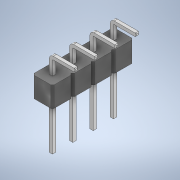
# Autodesk Inventor part: Part7
Saved by Autodesk Inventor 2021 (Build 250183000, 183)
## iProperties
Created: 2023-04-17
Part Number: Part7
Material: Generic
Document SubType Name: Modeling
Designer: stepa
Density: 1 g/cm^3
Appearance: Default
Author: stepa
Autodesk Inventor part; units mm, degrees
ref_plane "YZ Plane" through (0, 0, 0) normal (1, 0, 0) x (0, 1, 0)
ref_plane "XZ Plane" through (0, 0, 0) normal (0, 1, 0) x (-1, 0, 0)
sketch "Sketch1" plane through (0, 0, 0) normal (0, 1, 0) x (-1, 0, 0)
  line L0 (1.3038, 10.4024) -> (-0.7962, 10.4024)
  line L1 (-0.9962, 10.2024) -> (-0.9962, 8.1024)
  line L2 (-0.7962, 7.9024) -> (1.3038, 7.9024)
  line L3 (1.5038, 8.1024) -> (1.5038, 10.2024)
  line L4 (1.5038, 10.4024) -> (-0.9962, 7.9024) construction
  line L5 (-0.9962, 10.4024) -> (1.5038, 7.9024) construction
  line L6 (1.3038, 10.4024) -> (1.5038, 10.2024)
  line L7 (1.5038, 8.1024) -> (1.3038, 7.9024)
  line L8 (-0.9962, 8.1024) -> (-0.7962, 7.9024)
  line L9 (-0.9962, 10.2024) -> (-0.7962, 10.4024)
  line L10 (1.3038, 7.8624) -> (1.5038, 7.6624)
  line L11 (1.3038, 7.8624) -> (-0.7962, 7.8624)
  line L12 (-0.9962, 7.6624) -> (-0.7962, 7.8624)
  line L13 (1.5038, 5.5624) -> (1.5038, 7.6624)
  line L14 (1.5038, 5.5624) -> (1.3038, 5.3624)
  line L15 (-0.9962, 7.6624) -> (-0.9962, 5.5624)
  line L16 (-0.7962, 5.3624) -> (1.3038, 5.3624)
  line L17 (-0.9962, 5.5624) -> (-0.7962, 5.3624)
  line L18 (-0.9962, 7.8624) -> (1.5038, 5.3624) construction
  line L19 (1.5038, 7.8624) -> (-0.9962, 5.3624) construction
  line L20 (1.3038, 5.3224) -> (1.5038, 5.1224)
  line L21 (1.3038, 5.3224) -> (-0.7962, 5.3224)
  line L22 (-0.9962, 5.1224) -> (-0.7962, 5.3224)
  line L23 (1.5038, 3.0224) -> (1.5038, 5.1224)
  line L24 (1.5038, 3.0224) -> (1.3038, 2.8224)
  line L25 (-0.9962, 5.1224) -> (-0.9962, 3.0224)
  line L26 (-0.7962, 2.8224) -> (1.3038, 2.8224)
  line L27 (-0.9962, 3.0224) -> (-0.7962, 2.8224)
  line L28 (-0.9962, 5.3224) -> (1.5038, 2.8224) construction
  line L29 (1.5038, 5.3224) -> (-0.9962, 2.8224) construction
  line L30 (1.3038, 2.7824) -> (1.5038, 2.5824)
  line L31 (1.3038, 2.7824) -> (-0.7962, 2.7824)
  line L32 (-0.9962, 2.5824) -> (-0.7962, 2.7824)
  line L33 (1.5038, 0.4824) -> (1.5038, 2.5824)
  line L34 (1.5038, 0.4824) -> (1.3038, 0.2824)
  line L35 (-0.9962, 2.5824) -> (-0.9962, 0.4824)
  line L36 (-0.7962, 0.2824) -> (1.3038, 0.2824)
  line L37 (-0.9962, 0.4824) -> (-0.7962, 0.2824)
  line L38 (-0.9962, 2.7824) -> (1.5038, 0.2824) construction
  line L39 (1.5038, 2.7824) -> (-0.9962, 0.2824) construction
  line L40 (1.3038, 7.9024) -> (1.3038, 2.7824)
  line L41 (-0.7962, 2.7824) -> (-0.7962, 7.9024)
  point P0 (0, 0)
  point P1 (0.2538, 9.1524)
  point P2 (0.2538, 6.6124)
  point P3 (0.2538, 4.0724)
  point P4 (0.2538, 1.5324)
  dimension "d0" = 2.5
  dimension "d1" = 2.5
  dimension "d2" = 0.2
  dimension "d3" = 0.2
  dimension "d4" = 0.2
  dimension "d5" = 0.2
  dimension "d6" = 0.2
  dimension "d7" = 0.2
  dimension "d8" = 0.2
  dimension "d9" = 0.2
  dimension "d12" = 2.54
  constraints: 84 end point, 32 point on line, 8 midpoint, 2 parallel, 1 collinear, 1 horizontal, 1 perpendicular, 1 vertical, 68 other
  measures "d0" distance of L5.end L4.start
  measures "d1" distance of L4.end L5.end
  measures "d2" distance of L0.start L4.start
  measures "d3" distance of L3.end L4.start
  measures "d4" distance of L3.start L5.end
  measures "d5" distance of L2.end L5.end
  measures "d6" distance of L1.end L4.end
  measures "d7" distance of L2.start L4.end
  measures "d8" distance of L1.start L5.start
  measures "d9" distance of L0.end L5.start
  measures "d12" distance of L0.start L10.start
extrude "Extrusion1" add sketch "Sketch1" along normal blind 2.54
sketch "Sketch2" plane through (0, 2.54, 0) normal (0, 1, 0) x (1, 0, 0)
  line L0 (-1.5038, -8.1024) -> (-1.3038, -7.9024) projected
  line L1 (-1.3038, -7.9024) -> (-1.3038, -7.8624) projected
  line L2 (-1.3038, -7.8624) -> (-1.5038, -7.6624) projected
  line L3 (-1.5038, -7.6624) -> (-1.5038, -5.5624) projected
  line L4 (-1.5038, -5.5624) -> (-1.3038, -5.3624) projected
  line L5 (-1.3038, -5.3624) -> (-1.3038, -5.3224) projected
  line L6 (-1.3038, -5.3224) -> (-1.5038, -5.1224) projected
  line L7 (-1.5038, -5.1224) -> (-1.5038, -3.0224) projected
  line L8 (-1.5038, -3.0224) -> (-1.3038, -2.8224) projected
  line L9 (-1.3038, -2.8224) -> (-1.3038, -2.7824) projected
  line L10 (-1.3038, -2.7824) -> (-1.5038, -2.5824) projected
  line L11 (-1.5038, -2.5824) -> (-1.5038, -0.4824) projected
  line L12 (-1.5038, -0.4824) -> (-1.3038, -0.2824) projected
  line L13 (-1.3038, -0.2824) -> (0.7962, -0.2824) projected
  line L14 (0.7962, -0.2824) -> (0.9962, -0.4824) projected
  line L15 (0.9962, -0.4824) -> (0.9962, -2.5824) projected
  line L16 (0.9962, -2.5824) -> (0.7962, -2.7824) projected
  line L17 (0.7962, -2.7824) -> (0.7962, -2.8224) projected
  line L18 (0.7962, -2.8224) -> (0.9962, -3.0224) projected
  line L19 (0.9962, -3.0224) -> (0.9962, -5.1224) projected
  line L20 (0.9962, -5.1224) -> (0.7962, -5.3224) projected
  line L21 (0.7962, -5.3224) -> (0.7962, -5.3624) projected
  line L22 (0.7962, -5.3624) -> (0.9962, -5.5624) projected
  line L23 (0.9962, -5.5624) -> (0.9962, -7.6624) projected
  line L24 (0.9962, -7.6624) -> (0.7962, -7.8624) projected
  line L25 (0.7962, -7.8624) -> (0.7962, -7.9024) projected
  line L26 (0.7962, -7.9024) -> (0.9962, -8.1024) projected
  line L27 (0.9962, -8.1024) -> (0.9962, -10.2024) projected
  line L28 (0.9962, -10.2024) -> (0.7962, -10.4024) projected
  line L29 (0.7962, -10.4024) -> (-1.3038, -10.4024) projected
  line L30 (-1.3038, -10.4024) -> (-1.5038, -10.2024) projected
  line L31 (-1.5038, -10.2024) -> (-1.5038, -8.1024) projected
  point P0 (0, 0)
  point P1 (-0.2538, -1.5324)
  point P2 (-0.2538, -1.5324)
  point P3 (-0.2538, -4.0724)
  point P4 (-0.2538, -6.6124)
  point P5 (-0.2538, -9.1524)
  constraints: 1 coincident
ref_plane "Work Plane1" through (2.7462, 4.54, 9.1524) normal (1, 0, 0) x (0, 0, -1)
sketch "Sketch3" plane through (2.7462, 4.54, 9.1524) normal (1, 0, 0) x (0, 0, -1)
  line L0 (-0.2, 0.2) -> (0.2, 0.2)
  line L1 (0.2, 0.2) -> (0.2, -0.2)
  line L2 (0.2, -0.2) -> (-0.2, -0.2)
  line L3 (-0.2, -0.2) -> (-0.2, 0.2)
  line L4 (-0.2, 0.2) -> (0.2, -0.2) construction
  line L5 (0.2, 0.2) -> (-0.2, -0.2) construction
  line L6 (2.34, 0.2) -> (2.74, 0.2)
  line L7 (2.74, 0.2) -> (2.74, -0.2)
  line L8 (2.74, -0.2) -> (2.34, -0.2)
  line L9 (2.34, -0.2) -> (2.34, 0.2)
  line L10 (2.34, 0.2) -> (2.74, -0.2) construction
  line L11 (2.74, 0.2) -> (2.34, -0.2) construction
  line L12 (4.88, 0.2) -> (5.28, 0.2)
  line L13 (5.28, 0.2) -> (5.28, -0.2)
  line L14 (5.28, -0.2) -> (4.88, -0.2)
  line L15 (4.88, -0.2) -> (4.88, 0.2)
  line L16 (4.88, 0.2) -> (5.28, -0.2) construction
  line L17 (5.28, 0.2) -> (4.88, -0.2) construction
  line L18 (7.42, 0.2) -> (7.82, 0.2)
  line L19 (7.82, 0.2) -> (7.82, -0.2)
  line L20 (7.82, -0.2) -> (7.42, -0.2)
  line L21 (7.42, -0.2) -> (7.42, 0.2)
  line L22 (7.42, 0.2) -> (7.82, -0.2) construction
  line L23 (7.82, 0.2) -> (7.42, -0.2) construction
  point P0 (9.1524, -4.54)
  point P1 (0, 0)
  point P2 (2.54, 0)
  point P3 (5.08, 0)
  point P4 (7.62, 0)
  dimension "d32" = 0.4
  dimension "d33" = 0.4
  dimension "d36" = 2.54
  constraints: 48 end point, 8 midpoint, 2 horizontal, 2 parallel, 1 collinear, 1 perpendicular, 32 other
  measures "d32" distance of L0.end L1.end
  measures "d33" distance of L1.end L2.end
  measures "d36" distance of L0.start L6.start
sketch3d "3D Sketch2"
  line L0 (2.7462, 4.54, 9.1524) -> (0.0462, 4.54, 9.1524)
  arc A0 (0.0462, 4.54, 9.1524) -> (-0.2538, 4.24, 9.1524) centre (0.0462, 4.24, 9.1524) ccw
  line L1 (-0.2538, 4.24, 9.1524) -> (-0.2538, 2.54, 9.1524)
  dimension "d19" = 2
  dimension "d20" = 3
  dimension "d21" = 2
  dimension "d22" = 3
  dimension "d23" = 2
  dimension "d24" = 3
  dimension "d25" = 2
  dimension "d27" = 3
  dimension "d28" = 0.3
  dimension "d29" = 0.3
  dimension "d30" = 0.3
  dimension "d31" = 0.3
sweep "Sweep1" add profiles "Sketch3" path "3D Sketch2"
chamfer "Chamfer1" distance 0.1 angle 45 16 edges at (2.7462, 4.54, 9.3524) (2.7462, 4.74, 9.1524) (2.7462, 4.34, 9.1524) (2.7462, 4.54, 8.9524) (2.7462, 4.54, 6.8124) (2.7462, 4.74, 6.6124) (2.7462, 4.54, 6.4124) (2.7462, 4.34, 6.6124) (2.7462, 4.54, 4.2724) (2.7462, 4.74, 4.0724) (2.7462, 4.54, 3.8724) (2.7462, 4.34, 4.0724) (2.7462, 4.54, 1.7324) (2.7462, 4.74, 1.5324) (2.7462, 4.54, 1.3324) (2.7462, 4.34, 1.5324)
sketch "Sketch4" plane through (0, 0, 0) normal (0, -1, 0) x (1, 0, 0)
  line L0 (-1.3038, 7.9024) -> (-1.5038, 8.1024) projected
  line L1 (-1.5038, 8.1024) -> (-1.5038, 10.2024) projected
  line L2 (-1.5038, 10.2024) -> (-1.3038, 10.4024) projected
  line L3 (-1.3038, 10.4024) -> (0.7962, 10.4024) projected
  line L4 (0.7962, 10.4024) -> (0.9962, 10.2024) projected
  line L5 (0.9962, 10.2024) -> (0.9962, 8.1024) projected
  line L6 (0.9962, 8.1024) -> (0.7962, 7.9024) projected
  line L7 (0.7962, 7.9024) -> (0.7962, 7.8624) projected
  line L8 (0.7962, 7.8624) -> (0.9962, 7.6624) projected
  line L9 (0.9962, 7.6624) -> (0.9962, 5.5624) projected
  line L10 (0.9962, 5.5624) -> (0.7962, 5.3624) projected
  line L11 (0.7962, 5.3624) -> (0.7962, 5.3224) projected
  line L12 (0.7962, 5.3224) -> (0.9962, 5.1224) projected
  line L13 (0.9962, 5.1224) -> (0.9962, 3.0224) projected
  line L14 (0.9962, 3.0224) -> (0.7962, 2.8224) projected
  line L15 (0.7962, 2.8224) -> (0.7962, 2.7824) projected
  line L16 (0.7962, 2.7824) -> (0.9962, 2.5824) projected
  line L17 (0.9962, 2.5824) -> (0.9962, 0.4824) projected
  line L18 (0.9962, 0.4824) -> (0.7962, 0.2824) projected
  line L19 (0.7962, 0.2824) -> (-1.3038, 0.2824) projected
  line L20 (-1.3038, 0.2824) -> (-1.5038, 0.4824) projected
  line L21 (-1.5038, 0.4824) -> (-1.5038, 2.5824) projected
  line L22 (-1.5038, 2.5824) -> (-1.3038, 2.7824) projected
  line L23 (-1.3038, 2.7824) -> (-1.3038, 2.8224) projected
  line L24 (-1.3038, 2.8224) -> (-1.5038, 3.0224) projected
  line L25 (-1.5038, 3.0224) -> (-1.5038, 5.1224) projected
  line L26 (-1.5038, 5.1224) -> (-1.3038, 5.3224) projected
  line L27 (-1.3038, 5.3224) -> (-1.3038, 5.3624) projected
  line L28 (-1.3038, 5.3624) -> (-1.5038, 5.5624) projected
  line L29 (-1.5038, 5.5624) -> (-1.5038, 7.6624) projected
  line L30 (-1.5038, 7.6624) -> (-1.3038, 7.8624) projected
  line L31 (-1.3038, 7.8624) -> (-1.3038, 7.9024) projected
  line L32 (-0.0538, 1.3324) -> (-0.0538, 1.7324) projected
  line L33 (-0.4538, 1.3324) -> (-0.0538, 1.3324) projected
  line L34 (-0.4538, 1.7324) -> (-0.4538, 1.3324) projected
  line L35 (-0.0538, 1.7324) -> (-0.4538, 1.7324) projected
  line L36 (-0.4538, 3.8724) -> (-0.0538, 3.8724) projected
  line L37 (-1.5038, 8.1024) -> (-1.5038, 10.2024) projected
  line L38 (-1.3038, 7.9024) -> (-1.5038, 8.1024) projected
  line L39 (-1.3038, 7.8624) -> (-1.3038, 7.9024) projected
  line L40 (-1.5038, 7.6624) -> (-1.3038, 7.8624) projected
  line L41 (-1.5038, 5.5624) -> (-1.5038, 7.6624) projected
  line L42 (-1.3038, 5.3624) -> (-1.5038, 5.5624) projected
  line L43 (-1.3038, 5.3224) -> (-1.3038, 5.3624) projected
  line L44 (-1.5038, 5.1224) -> (-1.3038, 5.3224) projected
  line L45 (-1.5038, 3.0224) -> (-1.5038, 5.1224) projected
  line L46 (-1.3038, 2.8224) -> (-1.5038, 3.0224) projected
  line L47 (-1.3038, 2.7824) -> (-1.3038, 2.8224) projected
  line L48 (-1.5038, 2.5824) -> (-1.3038, 2.7824) projected
  line L49 (-1.5038, 0.4824) -> (-1.5038, 2.5824) projected
  line L50 (-1.3038, 0.2824) -> (-1.5038, 0.4824) projected
  line L51 (0.7962, 0.2824) -> (-1.3038, 0.2824) projected
  line L52 (0.9962, 0.4824) -> (0.7962, 0.2824) projected
  line L53 (0.9962, 2.5824) -> (0.9962, 0.4824) projected
  line L54 (0.7962, 2.7824) -> (0.9962, 2.5824) projected
  line L55 (0.7962, 2.8224) -> (0.7962, 2.7824) projected
  line L56 (0.9962, 3.0224) -> (0.7962, 2.8224) projected
  line L57 (0.9962, 5.1224) -> (0.9962, 3.0224) projected
  line L58 (0.7962, 5.3224) -> (0.9962, 5.1224) projected
  line L59 (0.7962, 5.3624) -> (0.7962, 5.3224) projected
  line L60 (0.9962, 5.5624) -> (0.7962, 5.3624) projected
  line L61 (0.9962, 7.6624) -> (0.9962, 5.5624) projected
  line L62 (0.7962, 7.8624) -> (0.9962, 7.6624) projected
  line L63 (0.7962, 7.9024) -> (0.7962, 7.8624) projected
  line L64 (0.9962, 8.1024) -> (0.7962, 7.9024) projected
  line L65 (0.9962, 10.2024) -> (0.9962, 8.1024) projected
  line L66 (0.7962, 10.4024) -> (0.9962, 10.2024) projected
  line L67 (-1.3038, 10.4024) -> (0.7962, 10.4024) projected
  line L68 (-1.5038, 10.2024) -> (-1.3038, 10.4024) projected
  line L69 (-0.4538, 4.2724) -> (-0.4538, 3.8724) projected
  line L70 (-0.0538, 4.2724) -> (-0.4538, 4.2724) projected
  line L71 (-0.0538, 3.8724) -> (-0.0538, 4.2724) projected
  line L72 (-0.0538, 6.8124) -> (-0.4538, 6.8124) projected
  line L73 (-0.4538, 6.8124) -> (-0.4538, 6.4124) projected
  line L74 (-0.4538, 6.4124) -> (-0.0538, 6.4124) projected
  line L75 (-0.0538, 6.4124) -> (-0.0538, 6.8124) projected
  line L76 (-0.0538, 8.9524) -> (-0.0538, 9.3524) projected
  line L77 (-0.0538, 9.3524) -> (-0.4538, 9.3524) projected
  line L78 (-0.4538, 9.3524) -> (-0.4538, 8.9524) projected
  line L79 (-0.4538, 8.9524) -> (-0.0538, 8.9524) projected
  point P0 (0, 0)
extrude "Extrusion2" add sketch "Sketch4" along normal blind 6 contours L33 L34 L35 L32 | L69 L70 L71 L36 | L75 L74 L73 L72 | L79 L78 L77 L76
chamfer "Chamfer2" distance 0.1 angle 45 16 edges at (-0.4538, -6, 9.1524) (-0.2538, -6, 9.3524) (-0.0538, -6, 9.1524) (-0.2538, -6, 8.9524) (-0.2538, -6, 6.8124) (-0.2538, -6, 6.4124) (-0.4538, -6, 6.6124) (-0.0538, -6, 6.6124) (-0.2538, -6, 4.2724) (-0.2538, -6, 3.8724) (-0.4538, -6, 4.0724) (-0.0538, -6, 4.0724) (-0.2538, -6, 1.7324) (-0.4538, -6, 1.5324) (-0.2538, -6, 1.3324) (-0.0538, -6, 1.5324)
equation "\"d5\" = d4"
equation "\"d6\" = d4"
equation "\"d7\" = d6"
equation "\"d8\" = d4"
equation "\"d9\" = d8"
equation "\"d30\" = d29"
equation "\"d31\" = d29"
body "Solid1"
